BioTrash Smell Absorber (Autodesk Fusion 360 design; units mm, degrees)
Autodesk Fusion 360 part; units mm, degrees
sketch "Sketch1" plane through (0, 0, 0) normal (0, 0, 1) x (1, 0, 0)
  line L0 (0, 0) -> (100, 0)
  line L1 (100, 0) -> (100, 100)
  line L2 (100, 100) -> (0, 100)
  line L3 (0, 100) -> (0, 0)
  line L4 (-2, -2) -> (102, -2)
  line L5 (102, -2) -> (102, 102)
  line L6 (102, 102) -> (-2, 102)
  line L7 (-2, 102) -> (-2, -2)
  line L8 (0, 75) -> (3, 75)
  line L9 (3, 75) -> (3, 73)
  line L10 (3, 73) -> (0, 73)
  line L11 (0, 73) -> (0, 75)
  line L12 (97, 25) -> (97, 27)
  line L13 (97, 27) -> (100, 27)
  line L14 (100, 25) -> (97, 25)
  line L15 (100, 27) -> (100, 25)
  line L16 (97, 73) -> (97, 75)
  line L17 (97, 75) -> (100, 75)
  line L18 (100, 73) -> (97, 73)
  line L19 (100, 75) -> (100, 73)
  line L20 (0, 25) -> (0, 27)
  line L21 (0, 27) -> (3, 27)
  line L22 (3, 25) -> (0, 25)
  line L23 (3, 27) -> (3, 25)
  line L24 (49, 97) -> (49, 100)
  line L25 (49, 100) -> (51, 100)
  line L26 (51, 97) -> (49, 97)
  line L27 (51, 100) -> (51, 97)
  line L28 (49, 0) -> (49, 3)
  line L29 (49, 3) -> (51, 3)
  line L30 (51, 0) -> (49, 0)
  line L31 (51, 3) -> (51, 0)
  dimension "d1" = 100
  dimension "d2" = 100
  dimension "d3" = 2
  dimension "d4" = 2
  dimension "d5" = 2
  dimension "d6" = 2
  dimension "d20" = 3
  dimension "d21" = 2
  dimension "d22" = 3
  dimension "d23" = 2
  dimension "d24" = 3
  dimension "d25" = 2
  dimension "d26" = 3
  dimension "d27" = 2
  dimension "d28" = 2
  dimension "d29" = 3
  dimension "d30" = 2
  dimension "d31" = 3
  dimension "d32" = 25
  dimension "d33" = 25
  dimension "d34" = 25
  dimension "d35" = 25
  dimension "d36" = 49
  dimension "d37" = 49
  constraint horizontal L0
  constraint vertical L1
  constraint horizontal L2
  constraint vertical L3
  constraint coincident L0.start L3.end
  constraint horizontal L4
  constraint vertical L5
  constraint horizontal L6
  constraint vertical L7
  constraint horizontal L8
  constraint vertical L9
  constraint horizontal L10
  constraint vertical L11
  constraint horizontal L13
  constraint vertical L15
  constraint horizontal L14
  constraint vertical L12
  constraint horizontal L17
  constraint vertical L19
  constraint horizontal L18
  constraint vertical L16
  constraint horizontal L21
  constraint vertical L23
  constraint horizontal L22
  constraint vertical L20
  constraint horizontal L25
  constraint vertical L27
  constraint horizontal L26
  constraint vertical L24
  constraint horizontal L29
  constraint vertical L31
  constraint horizontal L30
  constraint vertical L28
  constraint collinear L3 L11
  constraint collinear L3 L20
  constraint collinear L1 L19
  constraint collinear L1 L15
  constraint collinear L0 L30
  constraint collinear L2 L25
  measures "d1" distance of L0.start L0.end
  measures "d2" distance of L0.start L2.end
  measures "d3" distance of L2 L6
  measures "d4" distance of L1 L5
  measures "d5" distance of L0 L4
  measures "d6" distance of L3 L7
  measures "d20" distance of L8.start L8.end
  measures "d21" distance of L8.start L10.end
  measures "d22" distance of L13.end L12.end
  measures "d23" distance of L12.end L12.start
  measures "d24" distance of L17.end L16.end
  measures "d25" distance of L16.end L16.start
  measures "d26" distance of L21.end L20.end
  measures "d27" distance of L20.end L20.start
  measures "d28" distance of L25.end L24.end
  measures "d29" distance of L24.end L24.start
  measures "d30" distance of L29.end L28.end
  measures "d31" distance of L28.end L28.start
  measures "d32" distance of L2 L8
  measures "d33" distance of L0 L22
  measures "d34" distance of L2 L17
  measures "d35" distance of L0 L14
  measures "d36" distance of L3 L28
  measures "d37" distance of L3 L24
sketch "Sketch2" plane through (0, 0, 0) normal (0, 0, 1) x (1, 0, 0)
  circle A0 centre (10, 90) radius 5
  line L0 (100, 100) -> (0, 100)
  line L1 (0, 100) -> (0, 0)
  circle A1 centre (23.3333, 90) radius 5
  circle A2 centre (36.6667, 90) radius 5
  circle A3 centre (50, 90) radius 5
  circle A4 centre (63.3333, 90) radius 5
  circle A5 centre (76.6667, 90) radius 5
  circle A6 centre (90, 90) radius 5
  circle A7 centre (10, 76.6667) radius 5
  circle A8 centre (23.3333, 76.6667) radius 5
  circle A9 centre (36.6667, 76.6667) radius 5
  circle A10 centre (50, 76.6667) radius 5
  circle A11 centre (63.3333, 76.6667) radius 5
  circle A12 centre (76.6667, 76.6667) radius 5
  circle A13 centre (90, 76.6667) radius 5
  circle A14 centre (10, 63.3333) radius 5
  circle A15 centre (23.3333, 63.3333) radius 5
  circle A16 centre (36.6667, 63.3333) radius 5
  circle A17 centre (50, 63.3333) radius 5
  circle A18 centre (63.3333, 63.3333) radius 5
  circle A19 centre (76.6667, 63.3333) radius 5
  circle A20 centre (90, 63.3333) radius 5
  circle A21 centre (10, 50) radius 5
  circle A22 centre (23.3333, 50) radius 5
  circle A23 centre (36.6667, 50) radius 5
  circle A24 centre (50, 50) radius 5
  circle A25 centre (63.3333, 50) radius 5
  circle A26 centre (76.6667, 50) radius 5
  circle A27 centre (90, 50) radius 5
  circle A28 centre (10, 36.6667) radius 5
  circle A29 centre (23.3333, 36.6667) radius 5
  circle A30 centre (36.6667, 36.6667) radius 5
  circle A31 centre (50, 36.6667) radius 5
  circle A32 centre (63.3333, 36.6667) radius 5
  circle A33 centre (76.6667, 36.6667) radius 5
  circle A34 centre (90, 36.6667) radius 5
  circle A35 centre (10, 23.3333) radius 5
  circle A36 centre (23.3333, 23.3333) radius 5
  circle A37 centre (36.6667, 23.3333) radius 5
  circle A38 centre (50, 23.3333) radius 5
  circle A39 centre (63.3333, 23.3333) radius 5
  circle A40 centre (76.6667, 23.3333) radius 5
  circle A41 centre (90, 23.3333) radius 5
  circle A42 centre (10, 10) radius 5
  circle A43 centre (23.3333, 10) radius 5
  circle A44 centre (36.6667, 10) radius 5
  circle A45 centre (50, 10) radius 5
  circle A46 centre (63.3333, 10) radius 5
  circle A47 centre (76.6667, 10) radius 5
  circle A48 centre (90, 10) radius 5
  dimension "d7" = 10
  dimension "d8" = 10
  dimension "d9" = 10
  dimension "d12" = 80
  dimension "d13" = -80
  measures "d7" diameter of A0
  measures "d8" distance of A0.centre L0
  measures "d9" distance of A0.centre L1
extrude "Extrude1" add sketch "Sketch1" sketch "Sketch2" along normal blind 2 contours L0 L1 L2 L3 L8 L9 L10 L12 L13 L14 L16 L17 L18 L21 L22 L23 L24 L26 L27 L28 L29 L31 | L0 L28 L29 L30 L31 | L3 L20 L21 L22 L23 | L3 L8 L9 L10 L11 | L1 L12 L13 L14 L15 | L1 L16 L17 L18 L19 | L2 L24 L25 L26 L27 of sketch 2 contours A0 makes body 1
extrude "Extrude2" cut sketch "Sketch2" along normal blind 2 bodies 1
extrude "Extrude3" add sketch "Sketch1" along normal blind 12 contours L0 L28 L29 L30 L31 | L3 L20 L21 L22 L23 | L3 L8 L9 L10 L11 | L1 L12 L13 L14 L15 | L1 L16 L17 L18 L19 | L2 L24 L25 L26 L27 | L4 L5 L6 L7 bodies 1
sketch "Sketch3" plane through (0, 0, 12) normal (0, 0, 1) x (-1, 0, 0)
  line L0 (-51, 0) -> (-51, -3)
  line L1 (-51, -3) -> (-49, -3)
  line L2 (-49, -3) -> (-49, 0)
  line L3 (-49, 0) -> (0, 0)
  line L4 (0, 0) -> (0, -25)
  line L5 (0, -25) -> (-3, -25)
  line L6 (-3, -25) -> (-3, -27)
  line L7 (-3, -27) -> (0, -27)
  line L8 (0, -27) -> (0, -73)
  line L9 (0, -73) -> (-3, -73)
  line L10 (-3, -73) -> (-3, -75)
  line L11 (-3, -75) -> (0, -75)
  line L12 (0, -75) -> (0, -100)
  line L13 (0, -100) -> (-49, -100)
  line L14 (-49, -100) -> (-49, -97)
  line L15 (-49, -97) -> (-51, -97)
  line L16 (-51, -97) -> (-51, -100)
  line L17 (-51, -100) -> (-100, -100)
  line L18 (-100, -100) -> (-100, -75)
  line L19 (-100, -75) -> (-97, -75)
  line L20 (-97, -75) -> (-97, -73)
  line L21 (-97, -73) -> (-100, -73)
  line L22 (-100, -73) -> (-100, -27)
  line L23 (-100, -27) -> (-97, -27)
  line L24 (-97, -27) -> (-97, -25)
  line L25 (-97, -25) -> (-100, -25)
  line L26 (-100, -25) -> (-100, 0)
  line L27 (-100, 0) -> (-51, 0)
  line L28 (2, -102) -> (2, 2)
  line L29 (2, 2) -> (-102, 2)
  line L30 (-102, 2) -> (-102, -102)
  line L31 (-102, -102) -> (2, -102)
  line L32 (-37.5, -117) -> (-62.5, -117)
  line L33 (-62.5, -117) -> (-62.5, -102)
  line L34 (-62.5, -102) -> (-37.5, -102)
  line L35 (-37.5, -102) -> (-37.5, -117)
  line L36 (-102, -102) -> (2, -102)
  line L37 (0, -100) -> (0, 0)
  circle A0 centre (-50, -109.5) radius 1.5
  line L38 (-37.5, 2) -> (-62.5, 2)
  line L39 (-62.5, 2) -> (-62.5, 17)
  line L40 (-62.5, 17) -> (-37.5, 17)
  line L41 (-37.5, 17) -> (-37.5, 2)
  circle A1 centre (-50, 9.5) radius 1.5
  dimension "d38" = 25
  dimension "d39" = 15
  dimension "d40" = 37.5
  dimension "d41" = 3
  dimension "d46" = 25
  dimension "d47" = 15
  dimension "d48" = 37.5
  dimension "d49" = 3
  constraint horizontal L32
  constraint vertical L33
  constraint horizontal L34
  constraint vertical L35
  constraint collinear L34 L36
  constraint horizontal L38
  constraint vertical L39
  constraint horizontal L40
  constraint vertical L41
  constraint collinear L29 L38
  measures "d38" distance of L32.start L32.end
  measures "d39" distance of L32.start L34.end
  measures "d40" distance of L35 L37
  measures "d41" diameter of A0
  measures "d46" distance of L38.start L38.end
  measures "d47" distance of L38.start L40.end
  measures "d48" distance of L4 L41
  measures "d49" diameter of A1
extrude "Extrude4" add sketch "Sketch3" against normal blind 2 contours L31 L32 L33 L34 L35 L36 | L29 L38 L39 L40 L41 bodies 1
fillet "Fillet1" radius 9 2 edges at (62.5, 117, 11) (37.5, 117, 11) on bodies 1
fillet "Fillet1" radius 9 2 edges at (62.5, -17, 11) (37.5, -17, 11) on bodies 1
fillet "Fillet2" radius 4.5 1 edges at (50, 102, 10) on bodies 1
fillet "Fillet2" radius 4.5 1 edges at (50, -2, 10) on bodies 1
sketch "Sketch4" plane through (0, 0, 12) normal (0, 0, 1) x (-1, 0, 0)
  circle A0 centre (-50, 9.5) radius 1.5
  circle A1 centre (-50, -109.5) radius 1.5
  line L0 (-51, 0) -> (-51, -3)
  line L1 (-51, -3) -> (-49, -3)
  line L2 (-49, -3) -> (-49, 0)
  line L3 (-49, 0) -> (0, 0)
  line L4 (0, 0) -> (0, -25)
  line L5 (0, -25) -> (-3, -25)
  line L6 (-3, -25) -> (-3, -27)
  line L7 (-3, -27) -> (0, -27)
  line L8 (0, -27) -> (0, -73)
  line L9 (0, -73) -> (-3, -73)
  line L10 (-3, -73) -> (-3, -75)
  line L11 (-3, -75) -> (0, -75)
  line L12 (0, -75) -> (0, -100)
  line L13 (0, -100) -> (-49, -100)
  line L14 (-49, -100) -> (-49, -97)
  line L15 (-49, -97) -> (-51, -97)
  line L16 (-51, -97) -> (-51, -100)
  line L17 (-51, -100) -> (-100, -100)
  line L18 (-100, -100) -> (-100, -75)
  line L19 (-100, -75) -> (-97, -75)
  line L20 (-97, -75) -> (-97, -73)
  line L21 (-97, -73) -> (-100, -73)
  line L22 (-100, -73) -> (-100, -27)
  line L23 (-100, -27) -> (-97, -27)
  line L24 (-97, -27) -> (-97, -25)
  line L25 (-97, -25) -> (-100, -25)
  line L26 (-100, -25) -> (-100, 0)
  line L27 (-100, 0) -> (-51, 0)
  arc A2 (-37.5, 8) -> (-46.5, 17) centre (-46.5, 8) ccw
  line L28 (-46.5, 17) -> (-53.5, 17)
  arc A3 (-53.5, 17) -> (-62.5, 8) centre (-53.5, 8) ccw
  line L29 (-62.5, 8) -> (-62.5, 2)
  line L30 (-62.5, 2) -> (-102, 2)
  line L31 (-102, 2) -> (-102, -102)
  line L32 (-102, -102) -> (-62.5, -102)
  line L33 (-62.5, -102) -> (-62.5, -108)
  arc A4 (-62.5, -108) -> (-53.5, -117) centre (-53.5, -108) ccw
  line L34 (-53.5, -117) -> (-46.5, -117)
  arc A5 (-46.5, -117) -> (-37.5, -108) centre (-46.5, -108) ccw
  line L35 (-37.5, -108) -> (-37.5, -102)
  line L36 (-37.5, -102) -> (2, -102)
  line L37 (2, -102) -> (2, 2)
  line L38 (2, 2) -> (-37.5, 2)
  line L39 (-37.5, 2) -> (-37.5, 8)
  circle A6 centre (-50, -109.5) radius 1.5
  circle A7 centre (-50, 9.5) radius 1.5
  line L40 (-60, -114.5) -> (-40, -114.5)
  line L41 (-40, -114.5) -> (-40, -104.5)
  line L42 (-40, -104.5) -> (-60, -104.5)
  line L43 (-60, -104.5) -> (-60, -114.5)
  line L44 (-60, -114.5) -> (-40, -104.5) construction
  line L45 (-40, -114.5) -> (-60, -104.5) construction
  line L46 (-60, 14.5) -> (-40, 14.5)
  line L47 (-40, 14.5) -> (-40, 4.5)
  line L48 (-40, 4.5) -> (-60, 4.5)
  line L49 (-60, 4.5) -> (-60, 14.5)
  line L50 (-60, 14.5) -> (-40, 4.5) construction
  line L51 (-40, 14.5) -> (-60, 4.5) construction
  line L52 (-40, -104.5) -> (-60, -104.5)
  line L53 (-60, -104.5) -> (-60, 4.5)
  line L54 (-60, 4.5) -> (-40, 4.5)
  line L55 (-40, 4.5) -> (-40, -104.5)
  line L56 (-40, -104.5) -> (-60, -104.5)
  line L57 (-60, -104.5) -> (-60, -97)
  line L58 (-60, -97) -> (-40, -97)
  line L59 (-40, -97) -> (-40, -104.5)
  line L60 (-40, 4.5) -> (-60, 4.5)
  line L61 (-60, 4.5) -> (-60, -3)
  line L62 (-60, -3) -> (-40, -3)
  line L63 (-40, -3) -> (-40, 4.5)
  point P0 (-50, -109.5)
  point P1 (-50, 9.5)
  dimension "d52" = 20
  dimension "d53" = 10
  dimension "d54" = 20
  dimension "d55" = 10
  dimension "d56" = 20
  dimension "d57" = 7.5
  dimension "d58" = 20
  dimension "d59" = 7.5
  constraint concentric A1 A6
  constraint concentric A0 A7
  constraint horizontal L40
  constraint perpendicular L40 L41
  constraint parallel L40 L42
  constraint parallel L41 L43
  constraint coincident L44 P0
  constraint coincident L45 P0
  constraint coincident P0 A1.centre
  constraint horizontal L46
  constraint perpendicular L46 L47
  constraint parallel L46 L48
  constraint parallel L47 L49
  constraint coincident L50 P1
  constraint coincident L51 P1
  constraint coincident P1 A0.centre
  constraint horizontal L52
  constraint vertical L53
  constraint horizontal L54
  constraint vertical L55
  constraint horizontal L56
  constraint vertical L57
  constraint horizontal L58
  constraint vertical L59
  constraint horizontal L60
  constraint vertical L61
  constraint horizontal L62
  constraint vertical L63
  measures "d52" distance of L41.end L42.end
  measures "d53" distance of L40.end L41.end
  measures "d54" distance of L47.end L48.end
  measures "d55" distance of L46.end L47.end
  measures "d56" distance of L41.end L42.end
  measures "d57" distance of L41.end L58.end
  measures "d58" distance of L47.end L48.end
  measures "d59" distance of L47.end L62.end
extrude "Extrude5" add sketch "Sketch4" along normal blind 2 separate body contours A2 A3 L46 L47 L48 L49 L54 L60 | A3 L46 L49 | A2 L46 L47 | A4 A5 L40 L41 L42 L43 L52 L56 | A4 L40 L43 | A5 L40 L41 makes body 2 at (57.1667, -9.5, 12) makes body 3 at (42.8333, 109.5, 12)
extrude "Extrude6" add sketch "Sketch4" along normal blind 20 contours L0 L1 L2 L3 L27 L48 L53 L54 L55 L60 L61 L62 L63 | L0 L27 L53 L61 L62 | L2 L3 L55 L62 L63 | L16 L17 L53 L57 L58 | L13 L14 L55 L58 L59 | L13 L14 L15 L16 L17 L42 L52 L53 L55 L56 L57 L58 L59 bodies 2 3
extrude "Extrude7" add sketch "Sketch4" along normal blind 4 from surface at 16 contours L1 L15 L53 L55 L58 L62 bodies 2 3
fillet "Fillet3" radius 2 2 edges at (60, 50, 32) (40, 50, 32) on bodies 2
fillet "Fillet4" radius 2 2 edges at (60, 50, 28) (40, 50, 28) on bodies 2
fillet "Fillet5" radius 2 14 edges at (40, -4.5, 22) (40.5858, -4.5, 31.4142) (50, -4.5, 32) (59.4142, -4.5, 31.4142) (60, -4.5, 22) (40, 104.5, 22) (40.5858, 104.5, 31.4142) (50, 104.5, 32) (59.4142, 104.5, 31.4142) (60, 104.5, 22) (40, 97, 21) (40, 3, 21) (60, 97, 21) (60, 3, 21) on bodies 2
fillet "Fillet6" radius 3 4 edges at (40, -14.5, 13) (60, -14.5, 13) (40, 114.5, 13) (60, 114.5, 13) on bodies 2
hidden bodies 1
